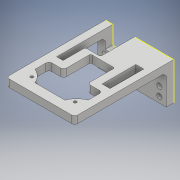
# Autodesk Inventor part: OpenMV-Mount-v2
Saved by Autodesk Inventor 2018.3 (Build 223284000, 284)
## iProperties
Created: 2019-03-21
Part Number: OpenMV-Mount-v2
Material: 一般
Document SubType Name: Modeling
Designer: shun2
Density: 1 g/cm^3
Appearance: 既定
Author: shun2
Autodesk Inventor part; units mm, degrees
ref_plane "YZ Plane" through (0, 0, 0) normal (1, 0, 0) x (0, 1, 0)
ref_plane "XZ Plane" through (0, 0, 0) normal (0, 1, 0) x (-1, 0, 0)
ref_plane "XY Plane" through (0, 0, 0) normal (0, 0, 1) x (1, 0, 0)
sketch "スケッチ1" plane through (0, 0, 0) normal (0, 0, 1) x (1, 0, 0)
  line L0 (-24.2059, 21.7891) -> (-24.2059, -29.3158)
  line L1 (-24.2059, -29.3158) -> (21.4201, -29.3158)
  line L2 (21.4196, -22.9707) -> (21.4201, -22.9707)
  line L3 (-11.4832, -22.9707) -> (8.6224, -22.9707)
  arc A0 (-11.4832, -22.9707) -> (-19.2289, -15.2115) centre (-24.2804, -28) ccw
  line L4 (-19.2289, -15.2115) -> (-19.2289, -7.8183)
  arc A1 (-17.2289, -5.8183) -> (-19.2289, -7.8183) centre (-17.2289, -7.8183) ccw
  line L5 (-17.2289, -5.8183) -> (-11.461, -5.8183)
  arc A2 (-11.461, -5.8183) -> (-9.461, -3.8183) centre (-11.461, -3.8183) ccw
  line L6 (-9.461, -3.8183) -> (-9.461, 11.1956)
  arc A3 (-8.461, 12.1956) -> (-9.461, 11.1956) centre (-8.461, 11.1956) ccw
  line L7 (-8.461, 12.1956) -> (5.6023, 12.1956)
  arc A4 (6.6023, 11.1956) -> (5.6023, 12.1956) centre (5.6023, 11.1956) ccw
  line L8 (6.6023, 11.1956) -> (6.6023, -3.8183)
  arc A5 (6.6023, -3.8183) -> (8.6023, -5.8183) centre (8.6023, -3.8183) ccw
  line L9 (8.6023, -5.8183) -> (14.3681, -5.8183)
  arc A6 (16.3681, -7.8183) -> (14.3681, -5.8183) centre (14.3681, -7.8183) ccw
  line L10 (16.3681, -7.8183) -> (16.3681, -15.2115)
  arc A7 (16.3681, -15.2115) -> (8.6224, -22.9707) centre (21.4196, -28) ccw
  circle A8 centre (13.0661, -20.6138) radius 0.954
  circle A9 centre (-15.8899, -20.6138) radius 0.954
  arc A10 (-13.9359, 14.1081) -> (-14.9359, 13.1081) centre (-13.9359, 13.1081) ccw
  line L11 (-14.9359, 13.1081) -> (-14.9359, -0.6888)
  line L12 (-14.9359, -0.6888) -> (-19.2289, -0.6888)
  arc A11 (-5.7797, 14.1081) -> (-4.7797, 15.1081) centre (-5.7797, 15.1081) ccw
  line L13 (-5.7797, 14.1081) -> (-13.9359, 14.1081)
  line L14 (-24.2059, 26.7891) -> (-24.2059, 21.7891)
  line L15 (21.4201, -29.3158) -> (-24.2059, -29.3158)
  line L16 (-24.2059, -29.3158) -> (-24.2059, 26.7891)
  line L17 (21.4196, 26.7891) -> (21.4201, 26.7891)
  line L18 (-24.2059, 36.7891) -> (-24.2059, 26.7891)
  line L19 (-19.2289, 36.7891) -> (-24.2059, 36.7891)
  line L20 (-19.2289, 36.7891) -> (-19.2289, -0.6888)
  line L21 (-4.7797, 15.1081) -> (-4.7797, 36.7891)
  line L22 (21.4201, -29.3158) -> (21.4201, 36.7891)
  line L23 (21.4201, 36.7891) -> (-4.7797, 36.7891)
  line L24 (11.6885, 21.2661) -> (16.9518, 21.2661)
  line L25 (16.9518, 21.2661) -> (16.9518, -1.2633)
  line L26 (16.9518, -1.2633) -> (11.6885, -1.2633)
  line L27 (11.6885, -1.2633) -> (11.6885, 21.2661)
  point P0 (0, 0)
  point P1 (0, 0)
  constraints: 56 end point, 20 point on circle, 12 centre point, 4 perpendicular, 3 parallel, 2 horizontal, 1 vertical
extrude "押し出し1" add sketch "スケッチ1" along normal blind 5
sketch "スケッチ2" plane through (0, 0, 0) normal (0, 0, -1) x (-1, 0, 0)
  line L0 (24.2059, 36.7891) -> (24.2059, -29.3158) projected
  line L1 (-21.4201, 36.7891) -> (24.2059, 36.7891)
  line L2 (24.2059, 36.7891) -> (24.2059, 31.7891)
  line L3 (24.2059, 31.7891) -> (-21.4201, 31.7891)
  line L4 (-21.4201, 31.7891) -> (-21.4201, 36.7891)
  point P0 (0, 0)
  dimension "d4" = 5
  constraints: 8 end point, 2 parallel, 1 horizontal, 1 perpendicular, 1 point on line
  measures "d4" distance of L1.end L2.end
extrude "押し出し2" add sketch "スケッチ2" along normal blind 20
sketch "スケッチ3" plane through (-4.7797, 36.7891, 5) normal (0, 1, 0) x (1, 0, 0)
  line L0 (-10.1561, 5) -> (-14.4492, 5) projected
  line L1 (-14.4492, 5) -> (0, 5)
  line L2 (0, 5) -> (0, 12)
  line L3 (0, 12) -> (-14.4492, 12)
  line L4 (-14.4492, 12) -> (-14.4492, 5)
  point P0 (4.7797, 5)
  dimension "d7" = 7
  constraints: 8 end point, 2 parallel, 1 horizontal, 1 perpendicular
  measures "d7" distance of L2.end L1.end
extrude "押し出し3" cut sketch "スケッチ3" against normal blind 20
sketch "スケッチ4" plane through (-4.7797, 36.7891, 5) normal (0, 1, 0) x (1, 0, 0)
  circle A0 centre (-14.9262, 21) radius 1.75
  line L0 (-19.4262, 25) -> (26.1998, 25) projected
  line L1 (-19.4262, 25) -> (-19.4262, 0) projected
  circle A1 centre (21.6998, 21) radius 1.75
  line L2 (26.1998, 25) -> (26.1998, 0) projected
  circle A2 centre (21.6998, 15) radius 1.75
  circle A3 centre (-14.9262, 15) radius 1.75
  point P0 (4.7797, 5)
  dimension "d10" = 3.5
  dimension "d11" = 4
  dimension "d12" = 4.5
  dimension "d13" = 3.5
  dimension "d14" = 4
  dimension "d15" = 4.5
  dimension "d16" = 3.5
  dimension "d17" = 6
  dimension "d18" = 3.5
  constraints: 4 centre point
  measures "d10" diameter of A0
  measures "d11" distance from line of L0 A0.centre
  measures "d12" distance from line of A0.centre L1
  measures "d13" diameter of A1
  measures "d14" distance from line of L0 A1.centre
  measures "d15" distance from line of L2 A1.centre
  measures "d16" diameter of A2
  measures "d17" distance of A1.centre A2.centre
  measures "d18" diameter of A3
fillet "フィレット1" radius 2 2 edges at (-24.2059, -29.3158, 2.5) (21.4201, -29.3158, 2.5)
extrude "押し出し4" cut sketch "スケッチ4" against normal blind 20
chamfer "面取り1" distance 2 angle 45 2 edges at (8.3202, 31.7891, 0) (-21.7174, 31.7891, 0)
sketch "スケッチ5" plane through (-4.7797, 36.7891, 5) normal (0, 1, 0) x (1, 0, 0)
  circle A0 centre (21.6998, 15) radius 1.75 projected
  circle A1 centre (-14.9262, 21) radius 1.75 projected
  circle A2 centre (21.6998, 21) radius 1.75 projected
  circle A3 centre (-14.9262, 15) radius 1.75 projected
  line L0 (-14.4492, 12) -> (-14.4492, 0) projected
  line L1 (-14.4492, 12) -> (0, 12) projected
  line L2 (0, 12) -> (0, 0) projected
  line L3 (26.1998, 0) -> (0, 0) projected
  line L4 (26.1998, 25) -> (26.1998, 0) projected
  line L5 (-19.4262, 25) -> (26.1998, 25) projected
  line L6 (-19.4262, 25) -> (-19.4262, 0) projected
  line L7 (-14.4492, 0) -> (-19.4262, 0) projected
  point P0 (4.7797, 5)
